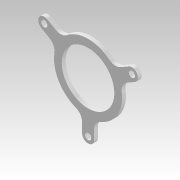
# Autodesk Inventor part: Bracket
Saved by Autodesk Inventor 2020 (Build 240168000, 168)
## iProperties
Created: 2022-01-15
Part Number: Bracket
Material: Generic
Document SubType Name: Modeling
Designer: DDeGo
Density: 1 g/cm^3
Appearance: Default
Author: DDeGo
Autodesk Inventor part; units mm, degrees
ref_plane "YZ Plane" through (0, 0, 0) normal (1, 0, 0) x (0, 1, 0)
ref_plane "XZ Plane" through (0, 0, 0) normal (0, 1, 0) x (-1, 0, 0)
ref_plane "XY Plane" through (0, 0, 0) normal (0, 0, 1) x (1, 0, 0)
sketch "Sketch1" plane through (0, 0, 0) normal (0, 0, 1) x (1, 0, 0)
  circle A0 centre (0, -30) radius 1.6
  circle A1 centre (0, 0) radius 13.5
  circle A2 centre (0, 0) radius 20
  line L0 (0, 0) -> (0, -30) construction
  line L1 (0, -30) -> (0, -7.0396) construction
  line L2 (-3.1, -30) -> (-3.1, -19.7583)
  arc A3 (-3.1, -30) -> (3.1, -30) centre (0, -30) ccw
  line L3 (3.1, -19.7583) -> (3.1, -30)
  circle A4 centre (25.9808, 15) radius 1.6
  line L4 (0, 0) -> (25.9808, 15) construction
  line L5 (25.9808, 15) -> (6.0965, 3.5198) construction
  line L6 (27.5308, 12.3153) -> (18.6612, 7.1945)
  arc A5 (27.5308, 12.3153) -> (24.4308, 17.6847) centre (25.9808, 15) ccw
  line L7 (15.5612, 12.5638) -> (24.4308, 17.6847)
  circle A6 centre (-25.9808, 15) radius 1.6
  line L8 (0, 0) -> (-25.9808, 15) construction
  line L9 (-25.9808, 15) -> (-6.0965, 3.5198) construction
  line L10 (-24.4308, 17.6847) -> (-15.5612, 12.5638)
  arc A7 (-24.4308, 17.6847) -> (-27.5308, 12.3153) centre (-25.9808, 15) ccw
  line L11 (-18.6612, 7.1945) -> (-27.5308, 12.3153)
  point P0 (18.6612, 7.1945)
  point P1 (15.5612, 12.5638)
  dimension "d4" = 30
  dimension "d5" = 3.2
  dimension "d6" = 27
  dimension "d7" = 40
  dimension "d8" = 1.5
  dimension "d11" = 360
  constraints: 30 end point, 8 centre point, 8 point on circle, 3 point on line, 2 coincident, 2 tangent, 2 vertical, 1 parallel, 40 other
  measures "d4" distance of L0.start L0.end
  measures "d5" diameter of A0
  measures "d6" diameter of A1
  measures "d7" diameter of A2
  measures "d8" radial gap between concentric circles of A0 A3
extrude "Extrusion1" add sketch "Sketch1" along normal blind 1.5
fillet "Fillet1" radius 5 6 edges at (-15.5612, 12.5638, 0.75) (15.5612, 12.5638, 0.75) (18.6612, 7.1945, 0.75) (-18.6612, 7.1945, 0.75) (-3.1, -19.7583, 0.75) (3.1, -19.7583, 0.75)
body "Solid1"
